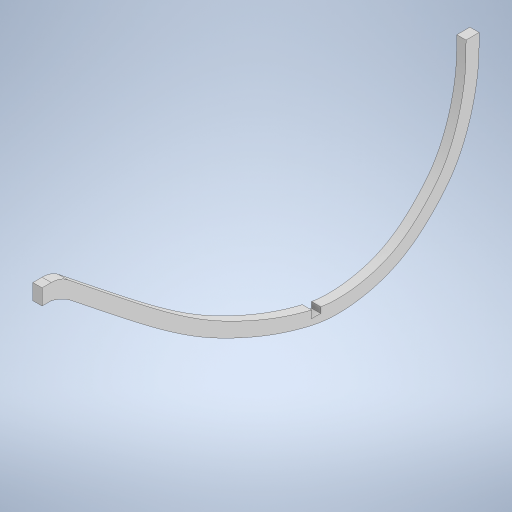
# Autodesk Inventor part: Balon skelet
Saved by Autodesk Inventor 2023 (Build 270158000, 158)
## iProperties
Created: 2022-12-16
Part Number: Balon skelet
Material: Generic
Document SubType Name: Modeling
Designer: David Zindović
Density: 1 g/cm^3
Appearance: Default
Author: David Zindović
Autodesk Inventor part; units mm, degrees
ref_plane "YZ Plane" through (0, 0, 0) normal (1, 0, 0) x (0, 1, 0)
ref_plane "XZ Plane" through (0, 0, 0) normal (0, 1, 0) x (-1, 0, 0)
ref_plane "XY Plane" through (0, 0, 0) normal (0, 0, 1) x (1, 0, 0)
sketch "Sketch1" plane through (0, 0, 0) normal (1, 0, 0) x (0, 1, 0)
  line L0 (0, 0) -> (-75, 0)
  line L1 (-75, 0) -> (-75, 160)
  line L2 (0, 160) -> (0, 0)
  line L3 (0, 56.3612) -> (0, 60.3607)
  line L4 (0, 0) -> (-10, 0)
  line L5 (-75.3991, 224.2517) -> (91.7561, 218.4145) construction
  line L6 (91.7561, 218.4145) -> (83.5776, -15.7872) construction
  line L7 (83.5776, -15.7872) -> (-83.5776, -9.95) construction
  line L8 (-83.5776, -9.95) -> (-75.3991, 224.2517) construction
  line L9 (-10, 0) -> (-17, 0) construction
  line L10 (-17, 0) -> (-23.6754, 0.353) construction
  line L11 (-23.6754, 0.353) -> (-32, 2) construction
  line L12 (-32, 2) -> (-39, 4) construction
  line L13 (-39, 4) -> (-49, 8) construction
  line L14 (-49, 8) -> (-57, 14) construction
  line L15 (-57, 14) -> (-65, 22) construction
  line L16 (-65, 22) -> (-70, 29) construction
  line L17 (-70, 29) -> (-74, 38) construction
  line L18 (-74, 38) -> (-76, 49) construction
  line L19 (-76, 49) -> (-76, 57) construction
  line L20 (-76, 57) -> (-75, 64) construction
  line L21 (-75, 64) -> (-71, 78) construction
  line L22 (-71, 78) -> (-65, 92) construction
  line L23 (-65, 92) -> (-57, 108) construction
  line L24 (-57, 108) -> (-47, 122) construction
  line L25 (-47, 122) -> (-37, 135) construction
  line L26 (-37, 135) -> (-17, 160) construction
  spline S0 degree 4 poles (-10, 0) (-17, 0) (-23.6754, 0.353) (-32, 2) (-39, 4) (-49, 8) (-57, 14) (-65, 22) (-70, 29) (-74, 38) (-76, 49) (-76, 57) (-75, 64) (-71, 78) (-65, 92) (-57, 108) (-47, 122) (-37, 135) (-17, 160) knots 1 1 1 1 1 2 3 4 5 6 7 8 9 10 11 12 13 14 15 16 16 16 16 16
  line L27 (0, -69) -> (-130, -69)
  line L28 (-10, 5) -> (0, 5)
  line L29 (-10, 0) -> (-10, 5)
  line L30 (-17, 160) -> (-11, 160) construction
  line L31 (0, 60.3607) -> (-70, 60.3607)
  line L32 (-70, 60.3607) -> (-70, 63.8607)
  line L33 (-70, 63.8607) -> (0, 63.8607)
  line L34 (0, 63.8607) -> (0, 60.3607)
  line L35 (-70, 60.3607) -> (-72.5, 60.3607)
  line L36 (-72.5, 60.3607) -> (-72.5, 63.8607)
  line L37 (-72.5, 63.8607) -> (-70, 63.8607)
  line L38 (-70, 63.8607) -> (-70, 60.3607)
  line L39 (0, 133.8805) -> (-30, 133.8805)
  line L40 (-30, 133.8805) -> (-30, 137.3805)
  line L41 (-30, 137.3805) -> (0, 137.3805)
  line L42 (0, 137.3805) -> (0, 133.8805)
  line L43 (-30, 137.3805) -> (-32.5, 137.3805)
  line L44 (-32.5, 137.3805) -> (-32.5, 133.8805)
  line L45 (-32.5, 133.8805) -> (-30, 133.8805)
  line L46 (-30, 133.8805) -> (-30, 137.3805)
  line L47 (-11, 160) -> (0, 160)
  line L48 (-13.1935, 156.7542) -> (-10.753, 160) construction
  line L49 (0, 160) -> (0, 163)
  arc A0 (-13.1935, 156.7542) -> (-11, 163) centre (-21.0107, 163.0077) ccw
  line L50 (-17, 160) -> (-17, 163) construction
  arc A1 (-20.9159, 155.1012) -> (-17, 163) centre (-37.16, 168.0744) ccw
  line L51 (-17, 163) -> (-11, 163)
  line L52 (-11, 163) -> (-17, 163)
  line L53 (-17, 163) -> (-17, 166.5)
  line L54 (-17, 166.5) -> (-11, 166.5)
  line L55 (-11, 166.5) -> (-11, 163)
  spline S1 degree 5 poles (-13.1935, 156.7541) (-18.3028, 150.3634) (-23.4151, 143.9741) (-28.4888, 137.5562) (-35.5181, 128.7265) (-42.2791, 119.6913) (-44.1018, 117.1812) (-47.258, 112.7293) (-50.2594, 108.172) (-51.5201, 106.1829) (-53.7905, 102.4259) (-55.9114, 98.5828) (-56.861, 96.7831) (-58.6188, 93.3248) (-60.2821, 89.8201) (-61.0536, 88.1444) (-62.5005, 84.904) (-63.8655, 81.6283) (-64.4986, 80.0462) (-65.6665, 76.9861) (-66.7379, 73.8909) (-67.2287, 72.3981) (-68.0807, 69.6659) (-68.8527, 66.9102) (-69.1835, 65.6628) (-69.7187, 63.5078) (-70.1667, 61.3332) (-70.3356, 60.4188) (-70.6006, 58.7126) (-70.7691, 56.9944) (-70.8249, 56.1996) (-70.8992, 54.5268) (-70.8879, 52.8522) (-70.8594, 51.9747) (-70.7491, 50.0729) (-70.5434, 48.1789) (-70.407, 47.1607) (-70.0771, 45.0707) (-69.6443, 42.9995) (-69.3935, 41.9398) (-68.8457, 39.8918) (-68.1752, 37.8809) (-67.8184, 36.9134) (-67.0679, 35.0711) (-66.2027, 33.2801) (-65.7597, 32.4303) (-64.8275, 30.7725) (-63.792, 29.1772) (-63.2532, 28.4023) (-62.0641, 26.7987) (-60.7869, 25.2641) (-60.0932, 24.472) (-58.6109, 22.8488) (-57.0649, 21.286) (-56.2445, 20.4865) (-54.603, 18.945) (-52.8993, 17.4727) (-52.0462, 16.7681) (-50.346, 15.4386) (-48.5677, 14.2158) (-47.6806, 13.6501) (-45.862, 12.5766) (-43.9787, 11.6211) (-43.0195, 11.1698) (-41.139, 10.3413) (-39.2258, 9.5917) (-38.293, 9.2453) (-36.4812, 8.6095) (-34.6478, 8.0393) (-33.7596, 7.7809) (-31.8597, 7.2634) (-29.9434, 6.8101) (-28.9234, 6.5865) (-26.6626, 6.1288) (-24.386, 5.7566) (-23.1356, 5.5791) (-19.7671, 5.1995) (-16.3786, 5.0524) (-14.2526, 5.018) (-12.1263, 4.9991) (-10, 5) knots 0 0 0 0 0 0 0.197163 0.197163 0.197163 0.271907 0.271907 0.271907 0.328638 0.328638 0.328638 0.37766 0.37766 0.37766 0.422109 0.422109 0.422109 0.463165 0.463165 0.463165 0.501025 0.501025 0.501025 0.532118 0.532118 0.532118 0.554517 0.554517 0.554517 0.573705 0.573705 0.573705 0.594853 0.594853 0.594853 0.619596 0.619596 0.619596 0.645824 0.645824 0.645824 0.670654 0.670654 0.670654 0.693732 0.693732 0.693732 0.716459 0.716459 0.716459 0.741821 0.741821 0.741821 0.769418 0.769418 0.769418 0.796069 0.796069 0.796069 0.821399 0.821399 0.821399 0.84693 0.84693 0.84693 0.870904 0.870904 0.870904 0.893189 0.893189 0.893189 0.918346 0.918346 0.918346 0.948764 0.948764 0.948764 1 1 1 1 1 1
  point P0 (0, -12.8686)
  point P1 (-70, 62.1107)
  point P2 (-70, 63.8607)
  point P3 (-69.6137, 63.8607)
  point P4 (-31.3772, 133.8805)
  point P5 (-28.619, 137.3805)
  point P6 (-75, 62.6097)
  point P7 (-75, 44.3417)
  point P8 (-70.3301, 60.3607)
  point P9 (-70, 62.1107)
  point P10 (-17, 163)
  dimension "d51" = 5
  dimension "d3" = 160
  dimension "d7" = 10
  dimension "d45" = 75
  dimension "d49" = 130
  dimension "d52" = 70
  dimension "d53" = 3.5
  dimension "d60" = 2.5
  dimension "d61" = 30
  dimension "d62" = 3.5
  dimension "d63" = 2.5
  dimension "d66" = 11
  dimension "d68" = 3
  dimension "d72" = 3.5
  constraints: 68 end point, 13 parallel, 8 horizontal, 7 perpendicular, 5 point on line, 4 point on circle, 2 centre point, 2 midpoint, 2 vertical, 2 vertical alignment, 1 collinear, 1 horizontal alignment, 12 other
  measures "d3" distance of L0.end L1.end
  measures "d7" distance of L0.start L4.end
  measures "d45" distance of L0.start L0.end
  measures "d49" distance of L27.start L27.end
  measures "d52" distance of L32.end L33.end
  measures "d53" distance of L31.end L32.end
  measures "d60" distance of L36.end L37.end
  measures "d61" distance of L40.end L41.end
  measures "d62" distance of L39.end L40.end
  measures "d63" distance of L45.end L44.end
  measures "d66" distance of L2.start L30.end
  measures "d68" distance of L2.start L49.end
  measures "d72" distance of L52.end L53.end
extrude "Extrusion1" add sketch "Sketch1" along normal mid plane 3.5 contours S0 L1 A1 L51 A0 S1 L41 L43 L44 L45 L33 L37 L36 L35 L29 | S0 L1 | L53 L54 L55 L51 | L45 L44 L43 L40 S1 | L40 L41 S1
body "Solid1"
